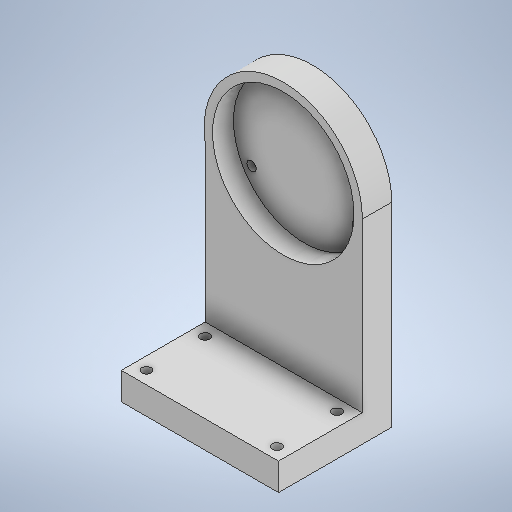
# Autodesk Inventor part: 电机支架-v0.1.0
Saved by Autodesk Inventor 2025 (Build 290162000, 162)
## iProperties
Created: 2025-05-07
Part Number: 电机支架-v0.1.0
Material: 常规
Document SubType Name: Modeling
Designer: hawav
Density: 1 g/cm^3
Appearance: 默认
Author: hawav
Autodesk Inventor part; units mm, degrees
ref_plane "YZ Plane" through (0, 0, 0) normal (1, 0, 0) x (0, 1, 0)
ref_plane "XZ Plane" through (0, 0, 0) normal (0, 1, 0) x (-1, 0, 0)
ref_plane "XY Plane" through (0, 0, 0) normal (0, 0, 1) x (1, 0, 0)
sketch "草图1" plane through (0, 0, 0) normal (0, 0, 1) x (1, 0, 0)
  circle A0 centre (0, 0) radius 33.75
  circle A1 centre (0, 0) radius 29
  circle A2 centre (0, 29) radius 2.25
  circle A3 centre (-25.1147, -14.5) radius 2.25
  circle A4 centre (25.1147, -14.5) radius 2.25
  circle A5 centre (0, 0) radius 37.75
  circle A6 centre (0, 0) radius 23.5
  dimension "d1" = 58
  dimension "d0" = 67.5
  dimension "d2" = 4.5
  dimension "d5" = 360
  dimension "d7" = 4
  dimension "d13" = 47
  constraints: 6 centre point, 3 coincident, 1 vertical alignment, 9 other
  measures "d0" diameter of A0
  measures "d2" diameter of A2
  measures "d7" radial gap between concentric circles of A0 A5
  measures "d13" diameter of A6
sketch "草图2" plane through (0, 0, 0) normal (0, 1, 0) x (-1, 0, 0)
  line L0 (37.75, 0) -> (-37.75, 0) projected
  line L1 (-37.75, 0) -> (37.25, 0)
  line L2 (37.25, 0) -> (37.25, 10)
  line L3 (37.25, 10) -> (-37.75, 10)
  line L4 (-37.75, 10) -> (-37.75, 0)
  line L5 (37.25, 0) -> (-37.75, 0)
  line L6 (-37.75, 0) -> (-37.75, -4)
  line L7 (-37.75, -4) -> (37.25, -4)
  line L8 (37.25, -4) -> (37.25, 0)
  point P0 (0, 0)
  dimension "d8" = 75
  dimension "d9" = 10
  dimension "d12" = 4
  constraints: 16 end point, 4 parallel, 2 horizontal, 2 perpendicular
  measures "d8" distance of L3.end L2.end
  measures "d9" distance of L2.end L1.end
  measures "d12" distance of L6.end L5.end
extrude "拉伸1" add sketch "草图2" against normal blind 80
extrude "拉伸2" cut sketch "草图1" along normal blind 10 contours A0 | A1 A4 A3 A2 | A2 A1 | A1 A2 | A4 A1 | A1 A4 | A3 A1 | A1 A3 | A6
extrude "拉伸3" cut sketch "草图1" against normal blind 10 contours A2 A1 | A1 A2 | A4 A1 | A1 A4 | A3 A1 | A1 A3
extrude "拉伸4" add sketch "草图1" against normal blind 4 contours A0 | A1 A4 A3 A2 | A5 | A6
extrude "拉伸5" add sketch "草图1" along normal blind 10 contours A5
sketch "草图3" plane through (0, -80, 0) normal (0, -1, 0) x (1, 0, 0)
  line L0 (-37.25, 10) -> (-37.25, -4) projected
  line L1 (-37.25, -4) -> (37.75, -4) projected
  line L2 (37.75, -4) -> (37.75, 10) projected
  line L3 (37.75, 10) -> (-37.25, 10) projected
  line L4 (37.75, 0) -> (-37.25, 0)
  line L5 (-37.25, 0) -> (-37.25, 50)
  line L6 (-37.25, 50) -> (37.75, 50)
  line L7 (37.75, 50) -> (37.75, 0)
  line L8 (37.75, -4) -> (-37.25, -4)
  line L9 (-37.25, -4) -> (-37.25, 0)
  line L10 (-37.25, 0) -> (37.75, 0)
  line L11 (37.75, 0) -> (37.75, -4)
  circle A0 centre (-31.25, 44) radius 2.25
  line L12 (0.25, 10) -> (0, 50)
  circle A1 centre (31.3226, 44.3911) radius 2.25
  line L13 (-37.25, 30) -> (37.75, 30)
  circle A2 centre (-31.25, 16) radius 2.25
  circle A3 centre (31.3226, 15.6089) radius 2.25
  point P0 (0, 0)
  dimension "d22" = 50
  dimension "d25" = 4.5
  dimension "d26" = 6
  dimension "d27" = 6
  constraints: 20 end point, 4 centre point, 4 parallel, 4 point on line, 3 perpendicular, 3 symmetric about line, 2 horizontal, 1 midpoint, 3 other
  measures "d22" distance of L4.end L5.end
  measures "d25" diameter of A0
  measures "d26" distance from line of L5 A0.centre
  measures "d27" distance from line of L6 A0.centre
extrude "拉伸6" add sketch "草图3" along normal blind 13
